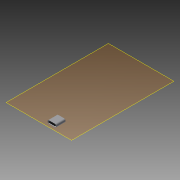
# Autodesk Inventor part: nanopc_t4_usb3c
Saved by Autodesk Inventor 2013 SP2 (Build 170200200, 200)
## iProperties
Created: 2018-09-03
Part Number: nanopc_t4_usb3c
Material: Generic
Document SubType Name: Modeling
Designer: alex
Density: 1 g/cm^3
Author: alex
Autodesk Inventor part; units mm, degrees
ref_plane "YZ Plane" through (0, 0, 0) normal (1, 0, 0) x (0, 1, 0)
ref_plane "XZ Plane" through (0, 0, 0) normal (0, 1, 0) x (-1, 0, 0)
ref_plane "XY Plane" through (0, 0, 0) normal (0, 0, 1) x (1, 0, 0)
ref_plane "Work Plane1" through (0, 0, 0) normal (0, 0, 1) x (1, 0, 0)
sketch "Sketch1" plane through (0, 0, 0) normal (0, 0, 1) x (1, 0, 0)
  line L0 (6.3465, -41.9537) -> (15.6465, -41.9537)
  line L1 (15.6465, -41.9537) -> (15.6465, -51.9537)
  line L2 (15.6465, -51.9537) -> (6.3465, -51.9537)
  line L3 (6.3465, -51.9537) -> (6.3465, -41.9537)
  point P0 (0, 0)
  dimension "d0" = 9.3
  dimension "d2" = 10
  constraints: 8 end point, 2 parallel, 1 horizontal, 1 perpendicular
  measures "d0" distance of L1.end L2.end
  measures "d2" distance of L0.end L1.end
extrude "Extrusion1" add sketch "Sketch1" along normal blind 3.5
fillet "Fillet1" radius 1.5 4 edges at (15.6465, -46.9537, 3.5) (6.3465, -46.9537, 3.5) (6.3465, -46.9537, 0) (15.6465, -46.9537, 0)
shell "Shell1" thickness 0.2 removed faces 1 at (9.9465, -51.9537, 2.3333)
sketch "Sketch2" plane through (7.8465, -42.1537, 3.3) normal (0, -1, 0) x (1, 0, 0)
  arc A0 (6.3, -3.1) -> (7.6, -1.8) centre (6.3, -1.8) ccw projected
  line L0 (7.6, -1.8) -> (7.6, -1.3) projected
  arc A1 (7.6, -1.3) -> (6.3, 0) centre (6.3, -1.3) ccw projected
  line L1 (6.3, 0) -> (0, 0) projected
  arc A2 (0, 0) -> (-1.3, -1.3) centre (0, -1.3) ccw projected
  line L2 (-1.3, -1.8) -> (-1.3, -1.3) projected
  arc A3 (-1.3, -1.8) -> (0, -3.1) centre (0, -1.8) ccw projected
  line L3 (0, -3.1) -> (6.3, -3.1) projected
  line L4 (0, -1.05) -> (6.3, -1.05)
  arc A4 (6.55, -1.3) -> (6.3, -1.05) centre (6.3, -1.3) ccw
  line L5 (6.55, -1.3) -> (6.55, -1.8)
  arc A5 (6.3, -2.05) -> (6.55, -1.8) centre (6.3, -1.8) ccw
  line L6 (6.3, -2.05) -> (0, -2.05)
  arc A6 (-0.25, -1.8) -> (0, -2.05) centre (0, -1.8) ccw
  line L7 (-0.25, -1.8) -> (-0.25, -1.3)
  arc A7 (0, -1.05) -> (-0.25, -1.3) centre (0, -1.3) ccw
  point P0 (-7.8465, -3.3)
  dimension "d7" = 1
  constraints: 8 end point, 8 point on circle, 4 centre point, 7 other
  measures "d7" distance between parallel lines of L6 L4
extrude "Extrusion2" add sketch "Sketch2" along normal up to surface (9.8 mm away) contours L4 A4 L5 A5 L6 A6 L7 A7
body "Solid1"
